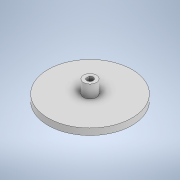
# Autodesk Inventor part: kolo
Saved by Autodesk Inventor 2020 (Build 240168000, 168)
## iProperties
Created: 2020-03-27
Part Number: kolo
Material: Generic
Document SubType Name: Modeling
Designer: Ondra
Density: 1 g/cm^3
Appearance: Default
Author: Ondra
Autodesk Inventor part; units mm, degrees
ref_plane "YZ Plane" through (0, 0, 0) normal (1, 0, 0) x (0, 1, 0)
ref_plane "XZ Plane" through (0, 0, 0) normal (0, 1, 0) x (-1, 0, 0)
ref_plane "XY Plane" through (0, 0, 0) normal (0, 0, 1) x (1, 0, 0)
sketch "Sketch1" plane through (0, 0, 0) normal (0, 1, 0) x (-1, 0, 0)
  circle A0 centre (0, 0) radius 32.5
  arc A1 (2, 1.5) -> (2, -1.5) centre (0, 0) ccw
  line L0 (-2.5, 0) -> (2, 0) construction
  line L1 (2, 0) -> (2, 1.5)
  line L2 (2, -1.5) -> (2, 0)
  dimension "d0" = 65
  constraints: 6 end point, 3 point on circle, 2 centre point, 2 coincident, 1 collinear, 1 horizontal, 1 point on line
  measures "d0" diameter of A0
extrude "Extrusion1" add sketch "Sketch1" along normal blind 5
sketch "Sketch2" plane through (0, 5, 0) normal (0, 1, 0) x (1, 0, 0)
  circle A0 centre (0, 0) radius 5
  arc A1 (-2, -1.5) -> (-2, 1.5) centre (0, 0) ccw projected
  arc A2 (-2, -1.5) -> (-2, 1.5) centre (0, 0) ccw
  line L0 (-2, -1.5) -> (-2, 1.5) projected
  line L1 (-2, -1.5) -> (-2, 1.5)
  dimension "d6" = 10
  constraints: 2 centre point, 2 coincident, 2 end point, 2 point on circle, 1 collinear
  measures "d6" diameter of A0
extrude "Extrusion2" add sketch "Sketch2" along normal blind 10
body "Solid1"
